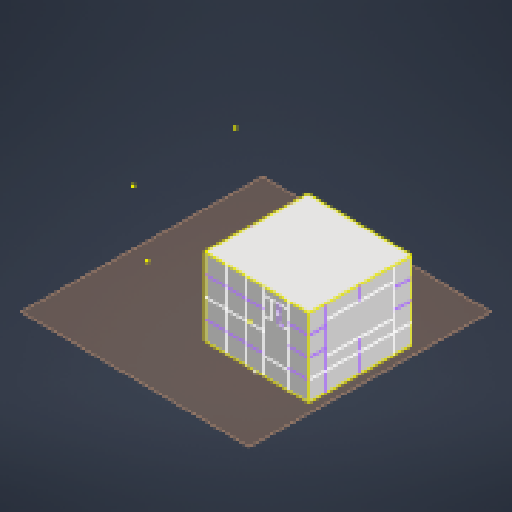
# Autodesk Inventor part: GeoReferencia
Saved by Autodesk Inventor 2024 (Build 280153000, 153)
## iProperties
Created: 2023-04-22
Part Number: GeoReferencia
Material: Genérico
Document SubType Name: Modeling
Designer: javie
Density: 1 g/cm^3
Appearance: Valor por defecto
Author: javie
Autodesk Inventor part; units mm, degrees
ref_plane "YZ Plane" through (0, 0, 0) normal (1, 0, 0) x (0, 1, 0)
ref_plane "XZ Plane" through (0, 0, 0) normal (0, 1, 0) x (-1, 0, 0)
ref_plane "XY Plane" through (0, 0, 0) normal (0, 0, 1) x (1, 0, 0)
ref_plane "Plano de trabajo1" through (2129.3345, -2770.6459, -3031.5298) normal (-0.0021155, 0.9999955, -0.0021345) x (-0.9998916, -0.0021464, -0.0145673)
sketch "Boceto1" plane through (2129.3345, -2770.6459, -3031.5298) normal (-0.0021155, 0.9999955, -0.0021345) x (-0.9998916, -0.0021464, -0.0145673)
  line L0 (0, 1445) -> (-3000, 1445)
  line L1 (-3000, 1445) -> (-3000, -1445)
  line L2 (-3000, -1445) -> (0, -1445)
  line L3 (0, -1445) -> (0, 1445)
  point P0 (2078.9955, 3068.0575)
  dimension "d0" = 3000
  dimension "d1" = 2890
  constraints: 8 end point, 2 parallel, 1 horizontal, 1 perpendicular
  measures "d0" distance of L2.end L1.end
  measures "d1" distance of L1.end L0.end
extrude "Extrusión1" add sketch "Boceto1" along normal blind 2200
sketch "Boceto2" plane through (5107.9529, -2761.1672, -1542.9845) normal (0.9998916, 0.0021464, 0.0145673) x (0.0145718, -0.0021035, -0.9998916)
  line L0 (0, 0) -> (0, 2200) projected
  line L1 (0, 550) -> (2890, 550)
  line L2 (2890, 0) -> (2890, 2200) projected
  line L3 (0, 2200) -> (2890, 2200) projected
  line L4 (0, 0) -> (2890, 0) projected
  line L5 (2390, 2200) -> (2390, 0)
  line L6 (500, 1800) -> (2390, 1800)
  line L7 (2390, 900) -> (500, 900)
  line L8 (1445, 2200) -> (1445, 1800)
  line L9 (1445, 900) -> (1445, 0)
  line L10 (2890, 1100) -> (2390, 1100)
  line L11 (500, 1100) -> (0, 1100)
  line L12 (0, 1650) -> (500, 1650)
  line L13 (2390, 1650) -> (2890, 1650)
  line L14 (2390, 1100) -> (2390, 900)
  line L15 (500, 0) -> (500, 2200)
  point P0 (-1623.0575, 2768.6672)
  dimension "d6" = 550
  dimension "d8" = 500
  dimension "d10" = 900
  dimension "d11" = 900
  constraints: 24 end point, 9 point on line, 6 midpoint, 6 perpendicular, 4 horizontal, 1 parallel, 1 vertical
  measures "d6" distance between parallel lines of L4 L1
  measures "d8" distance between parallel lines of L2 L5
  measures "d10" distance between parallel lines of L4 L7
  measures "d11" distance between parallel lines of L6 L7
sketch "Boceto3" plane through (5150.0655, -2767.2462, -4432.6713) normal (0.0145718, -0.0021035, -0.9998916) x (-0.9998916, -0.0021464, -0.0145673)
  line L0 (0, 0) -> (0, 2200) projected
  line L1 (3000, 0) -> (3000, 2200) projected
  line L2 (0, 2200) -> (3000, 2200) projected
  line L3 (2400, 2200) -> (2400, 0)
  line L4 (0, 0) -> (3000, 0) projected
  line L5 (1800, 2200) -> (1800, 0)
  line L6 (1300, 2200) -> (1300, 0)
  line L7 (600, 2200) -> (600, 0)
  line L8 (600, 1995) -> (1300, 1995)
  line L9 (870, 1995) -> (870, 1495)
  line L10 (870, 1495) -> (600, 1495)
  line L11 (1070, 1995) -> (1070, 1495)
  line L12 (1070, 1495) -> (1300, 1495)
  line L13 (600, 495) -> (1300, 495)
  line L14 (0, 1650) -> (600, 1650)
  line L15 (1300, 1650) -> (3000, 1650)
  line L16 (0, 550) -> (600, 550)
  line L17 (1300, 550) -> (3000, 550)
  line L18 (0, 1100) -> (600, 1100)
  line L19 (1300, 1100) -> (3000, 1100)
  point P0 (5078.9955, 2768.6672)
  dimension "d15" = 600
  dimension "d16" = 600
  dimension "d17" = 600
  dimension "d18" = 500
  dimension "d19" = 500
  dimension "d20" = 200
  dimension "d21" = 230
  dimension "d22" = 1000
  dimension "d23" = 205
  constraints: 32 end point, 26 point on line, 6 perpendicular, 4 horizontal, 3 parallel, 2 midpoint, 2 vertical
  measures "d15" distance between parallel lines of L0 L7
  measures "d16" distance between parallel lines of L1 L3
  measures "d17" distance between parallel lines of L3 L5
  measures "d18" distance between parallel lines of L5 L6
  measures "d19" distance of L9.start L9.end
  measures "d20" distance between parallel lines of L11 L9
  measures "d21" distance between parallel lines of L6 L11
  measures "d22" distance between parallel lines of L13 L10
  measures "d23" distance between parallel lines of L2 L8
sketch "Boceto4" plane through (2108.2782, -2767.6064, -1586.6864) normal (-0.0145718, 0.0021035, 0.9998916) x (0.9998916, 0.0021464, 0.0145673)
  line L0 (3000, 2200) -> (0, 2200) projected
  line L1 (600, 2200) -> (600, 0)
  line L2 (3000, 0) -> (0, 0) projected
  line L3 (1200, 2200) -> (1200, 0)
  line L4 (1700, 2200) -> (1700, 0)
  line L5 (2400, 2200) -> (2400, 0)
  line L6 (0, 0) -> (0, 2200) projected
  line L7 (3000, 0) -> (3000, 2200) projected
  line L8 (0, 0) -> (0, 2200) projected
  line L9 (1700, 1995) -> (2400, 1995)
  line L10 (1930, 1995) -> (1930, 1495)
  line L11 (1930, 1495) -> (1700, 1495)
  line L12 (2130, 1995) -> (2130, 1495)
  line L13 (2130, 1495) -> (2400, 1495)
  line L14 (0, 1650) -> (1700, 1650)
  line L15 (2400, 1650) -> (3000, 1650)
  line L16 (0, 1100) -> (1700, 1100)
  line L17 (2400, 1100) -> (3000, 1100)
  line L18 (0, 550) -> (1700, 550)
  line L19 (2400, 550) -> (3000, 550)
  line L20 (1700, 495) -> (2400, 495)
  point P0 (-2078.9955, 2768.6672)
  point P1 (2130, 1745)
  point P2 (2265, 1495)
  point P3 (1500, 0)
  dimension "d24" = 600
  dimension "d25" = 600
  dimension "d26" = 500
  dimension "d27" = 600
  dimension "d31" = 500
  dimension "d33" = 205
  dimension "d34" = 230
  dimension "d35" = 200
  dimension "d36" = 1000
  dimension "d46" = 495
  dimension "d47" = 1100
  constraints: 32 end point, 24 point on line, 11 perpendicular, 7 midpoint, 2 vertical, 1 horizontal
  measures "d24" distance between parallel lines of L1 L6
  measures "d25" distance between parallel lines of L3 L1
  measures "d26" distance between parallel lines of L4 L3
  measures "d27" distance between parallel lines of L7 L5
  measures "d31" distance of L10.start L10.end
  measures "d33" distance between parallel lines of L0 L9
  measures "d34" distance between parallel lines of L4 L10
  measures "d35" distance from line of point (2130, 1745) L10
  measures "d36" distance from line of L20 point (2265, 1495)
  measures "d46" distance between parallel lines of L2 L20
  measures "d47" distance from line of point (1500, 0) L16
sketch "Boceto5" plane through (2150.3908, -2773.6854, -4476.3732) normal (-0.9998916, -0.0021464, -0.0145673) x (-0.0145718, 0.0021035, 0.9998916)
  line L0 (2890, 0) -> (0, 0) projected
  line L1 (2090, 0) -> (2090, 1800)
  line L2 (2890, 2200) -> (0, 2200) projected
  line L3 (2090, 1800) -> (2890, 1800)
  line L4 (2890, 0) -> (2890, 2200) projected
  line L5 (2090, 1800) -> (2090, 2200)
  line L6 (0, 0) -> (0, 2200) projected
  line L7 (0, 1700) -> (2090, 1700)
  line L8 (0, 800) -> (2090, 800)
  line L9 (200, 1700) -> (200, 800)
  line L10 (1890, 1700) -> (1890, 800)
  line L11 (500, 2200) -> (500, 1700)
  line L12 (500, 800) -> (500, 0)
  line L13 (1590, 2200) -> (1590, 1700)
  line L14 (1590, 800) -> (1590, -24.3728)
  point P0 (4513.0575, 2768.6672)
  point P1 (2090, 2000)
  dimension "d37" = 1800
  dimension "d38" = 800
  dimension "d39" = 800
  dimension "d40" = 500
  dimension "d44" = 200
  dimension "d45" = 200
  constraints: 22 end point, 17 point on line, 11 perpendicular, 1 midpoint
  measures "d37" distance of L1.start L1.end
  measures "d38" distance between parallel lines of L4 L1
  measures "d39" distance between parallel lines of L0 L8
  measures "d40" distance between parallel lines of L2 L7
  measures "d44" distance between parallel lines of L6 L9
  measures "d45" distance between parallel lines of L1 L10
